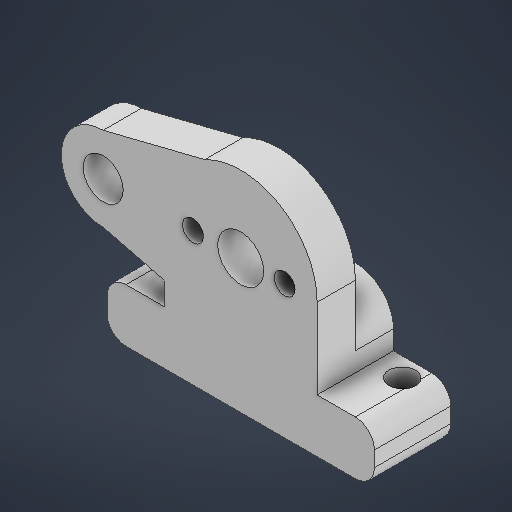
# Autodesk Inventor part: suportCaptor
Saved by Autodesk Inventor 2026.1 (Build 301233000, 233)
## iProperties
Created: 2026-01-27
Part Number: suportCaptor
Material: Generic
Document SubType Name: Modeling
Designer: fheli
Density: 1 g/cm^3
Appearance: Default
Author: fheli
Autodesk Inventor part; units mm, degrees
ref_plane "YZ Plane" through (0, 0, 0) normal (1, 0, 0) x (0, 1, 0)
ref_plane "XZ Plane" through (0, 0, 0) normal (0, 1, 0) x (-1, 0, 0)
ref_plane "XY Plane" through (0, 0, 0) normal (0, 0, 1) x (1, 0, 0)
sketch "Sketch1" plane through (0, 0, 0) normal (0, 0, 1) x (1, 0, 0)
  circle A0 centre (0, 0) radius 20
  circle A1 centre (0, 0) radius 6
  line L0 (0, 0) -> (-12.5, 0)
  line L1 (0, 0) -> (11.5, 0)
  circle A2 centre (-12.5, 0) radius 2.75
  circle A3 centre (11.5, 0) radius 2.75
  line L2 (0, 0) -> (-36, 0)
  circle A4 centre (-36, 0) radius 5.25
  circle A5 centre (-36, 0) radius 11
  line L3 (-36, 11) -> (0, 20)
  line L4 (-36, -11) -> (0, -20)
  line L5 (20, 0) -> (-20, 0)
  line L6 (-20, 0) -> (-20, 20)
  line L7 (-20, 20) -> (20, 20)
  line L8 (20, 20) -> (20, 0)
  line L9 (-20, 0) -> (20, 0)
  line L10 (20, 0) -> (20, -35)
  line L11 (20, -35) -> (-20, -35)
  line L12 (-20, -35) -> (-20, 0)
  point P0 (-9.4118, -17.6471)
  point P1 (-9.4118, 17.6471)
  point P2 (-20, -15)
  dimension "d0" = 40
  dimension "d1" = 12
  dimension "d2" = 12.5
  dimension "d3" = 11.5
  dimension "d4" = 5.5
  dimension "d5" = 5.5
  dimension "d8" = 36
  dimension "d9" = 10.5
  dimension "d10" = 22
  dimension "d11" = 40
  dimension "d12" = 20
  dimension "d13" = 40
  dimension "d14" = 35
  constraints: 26 end point, 6 centre point, 6 coincident, 5 horizontal, 5 point on circle, 4 parallel, 2 perpendicular
  measures "d0" diameter of A0
  measures "d1" diameter of A1
  measures "d2" distance of L0.start L0.end
  measures "d3" distance of L0.start L1.end
  measures "d4" diameter of A2
  measures "d5" diameter of A3
  measures "d8" distance of L0.start L2.end
  measures "d9" diameter of A4
  measures "d10" diameter of A5
  measures "d11" distance of L6.end L7.end
  measures "d12" distance of L5.end L6.end
  measures "d13" distance of L10.end L11.end
  measures "d14" distance of L9.end L10.end
extrude "Extrusion1" add sketch "Sketch1" along normal blind 10 contours L5 A3 L1 A1 L0 A2 L2 A0 L3 | L10 L11 L12 L4 A0 | A0 L4 L2 A2 L0 A1 L1 A3 L5 | L3 A0 | A0 L4 | A0 L6 L3 | L4 L12 A0 | L12 L4 A5 L2 | L2 A5 L3 L6 | A5
sketch "Sketch3" plane through (0, 0, 0) normal (0, 0, -1) x (-1, 0, 0)
  line L0 (-20, -35) -> (-20, 0) projected
  line L1 (-20, -35) -> (20, -35)
  line L2 (20, -35) -> (20, -6)
  line L3 (20, -6) -> (-20, -6)
  line L4 (-20, -6) -> (-20, -35)
  point P0 (0, 0)
  point P1 (-20, -6)
  dimension "d15" = 40
  dimension "d16" = 29
  constraints: 8 end point, 2 parallel, 1 horizontal, 1 perpendicular
  measures "d15" distance of L3.end L2.end
  measures "d16" distance of L2.end L1.end
extrude "Extrusion2" add sketch "Sketch3" along normal blind 10
fillet "Fillet3" radius 10 1 edges at (-20, -6, -5)
fillet "Fillet4" radius 10 1 edges at (20, -6, -5)
sketch "Sketch4" plane through (20, -35, 10) normal (1, 0, 0) x (0, 0, -1)
  line L0 (20, 0) -> (0, 0) projected
  line L1 (0, 0) -> (20, 0)
  line L2 (20, 0) -> (20, 14)
  line L3 (20, 14) -> (0, 14)
  line L4 (0, 14) -> (0, 0)
  point P0 (10, 35)
  dimension "d23" = 20
  dimension "d24" = 14
  constraints: 8 end point, 2 parallel, 1 horizontal, 1 perpendicular
  measures "d23" distance of L3.end L2.end
  measures "d24" distance of L2.end L1.end
extrude "Extrusion3" add sketch "Sketch4" along normal blind 15
sketch "Sketch5" plane through (-20, -35, -10) normal (-1, 0, 0) x (0, 0, 1)
  line L0 (0, 0) -> (0, 14) projected
  line L1 (20, 14) -> (20, 0) projected
  line L2 (0, 0) -> (20, 0)
  line L3 (20, 0) -> (20, 14)
  line L4 (20, 14) -> (0, 14)
  line L5 (0, 14) -> (0, 0)
  point P0 (10, 35)
  dimension "d27" = 20
  constraints: 8 end point, 2 parallel, 1 horizontal, 1 perpendicular
  measures "d27" distance of L4.end L1.start
extrude "Extrusion4" add sketch "Sketch5" along normal blind 15
sketch "Sketch6" plane through (-20, -21, 10) normal (0, 1, 0) x (1, 0, 0)
  circle A0 centre (-7.5, 15) radius 3.5
  point P0 (20, 10)
  dimension "d30" = 7
  constraints: 1 centre point
  measures "d30" diameter of A0
sketch "Sketch7" plane through (20, -21, 10) normal (0, 1, 0) x (1, 0, 0)
  circle A0 centre (7.273, 15) radius 3.5
  point P0 (-20, 10)
  dimension "d31" = 7
  constraints: 1 centre point
  measures "d31" diameter of A0
extrude "Extrusion5" cut sketch "Sketch7" against normal blind 15
extrude "Extrusion6" cut sketch "Sketch6" against normal blind 15
fillet "Fillet5" radius 5 1 edges at (35, -35, 0)
fillet "Fillet6" radius 5 1 edges at (35, -21, 0)
fillet "Fillet7" radius 5 1 edges at (-35, -35, 0)
fillet "Fillet8" radius 5 1 edges at (-35, -21, 0)
body "Solid1"
